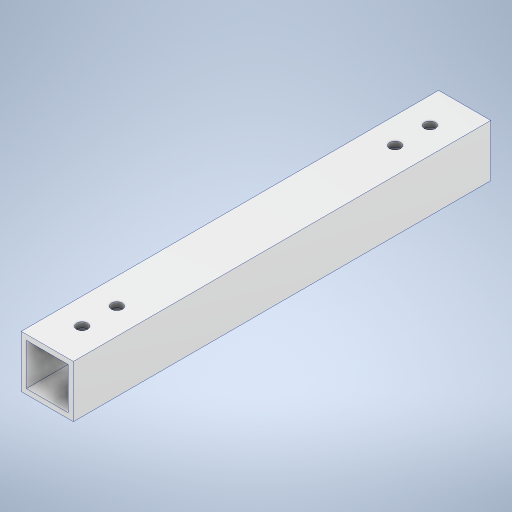
# Autodesk Inventor part: 射出_角柱9
Saved by Autodesk Inventor 2023 (Build 270158000, 158)
## iProperties
Created: 2022-04-20
Part Number: 射出_角柱9
Material: アルミニウム 6061
Document SubType Name: Modeling
Designer: yuta
Density: 2.7 g/cm^3
Appearance: アルミニウム - フラット
Author: yuta
Autodesk Inventor part; units mm, degrees
ref_plane "YZ Plane" through (0, 0, 0) normal (1, 0, 0) x (0, 1, 0)
ref_plane "XZ Plane" through (0, 0, 0) normal (0, 1, 0) x (-1, 0, 0)
ref_plane "XY Plane" through (0, 0, 0) normal (0, 0, 1) x (1, 0, 0)
sketch "スケッチ1" plane through (0, 0, 0) normal (0, 0, 1) x (1, 0, 0)
  line L0 (0, 0) -> (15, 0)
  line L1 (15, 0) -> (15, 15)
  line L2 (15, 15) -> (0, 15)
  line L3 (0, 15) -> (0, 0)
  dimension "d0" = 15
  dimension "d1" = 15
  constraints: 8 end point, 2 parallel, 1 horizontal, 1 perpendicular
  measures "d0" distance of L2.end L1.end
  measures "d1" distance of L1.end L0.end
extrude "押し出し1" add sketch "スケッチ1" along normal blind 120
sketch "スケッチ2" plane through (0, 15, 0) normal (0, 1, 0) x (1, 0, 0)
  line L0 (0, 0) -> (0, -120) projected
  line L1 (15, 0) -> (0, 0) projected
  line L2 (15, -120) -> (0, -120) projected
  point P0 (7.5, -10)
  point P1 (7.5, -20)
  point P2 (7.5, -110)
  point P3 (7.5, -100)
  dimension "d4" = 7.5
  dimension "d5" = 10
  dimension "d6" = 10
  dimension "d7" = 7.5
  dimension "d8" = 10
  dimension "d9" = 7.5
  dimension "d10" = 10
  dimension "d11" = 7.5
  measures "d4" distance from line of L0 point (7.5, -10)
  measures "d5" distance from line of L1 point (7.5, -10)
  measures "d6" distance of point (7.5, -20) point (7.5, -10)
  measures "d7" distance from line of L0 point (7.5, -20)
  measures "d8" distance from line of L2 point (7.5, -110)
  measures "d9" distance from line of L0 point (7.5, -110)
  measures "d10" distance of point (7.5, -110) point (7.5, -100)
  measures "d11" distance from line of L0 point (7.5, -100)
hole "穴1" at (7.5, 15, 10) at (7.5, 15, 20) at (7.5, 15, 110) at (7.5, 15, 100) direction (0, -1, 0) diameter 3.2 end through all
sketch "スケッチ3" plane through (0, 0, 120) normal (0, 0, 1) x (1, 0, 0)
  line L0 (1.5, 13.5) -> (13.5, 13.5)
  line L1 (13.5, 13.5) -> (13.5, 1.5)
  line L2 (13.5, 1.5) -> (1.5, 1.5)
  line L3 (1.5, 1.5) -> (1.5, 13.5)
  line L4 (15, 15) -> (0, 15) projected
  line L5 (0, 15) -> (0, 0) projected
  dimension "d19" = 12
  dimension "d20" = 12
  dimension "d21" = 1.5
  dimension "d22" = 1.5
  constraints: 8 end point, 2 parallel, 1 horizontal, 1 perpendicular
  measures "d19" distance of L1.end L2.end
  measures "d20" distance of L0.end L1.end
  measures "d21" distance between parallel lines of L4 L0
  measures "d22" distance between parallel lines of L5 L3
extrude "押し出し2" cut sketch "スケッチ3" against normal blind 200
